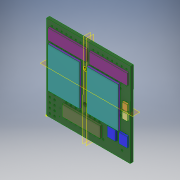
# Autodesk Inventor part: NixieModule_IN12.brd
Saved by Autodesk Inventor 2019 (Build 230136000, 136)
## iProperties
Created: 2019-08-02
Part Number: NixieModule_IN12.brd
Material: Generisch
Document SubType Name: Modeling
Designer: grubi
Density: 1 g/cm^3
Appearance: Board-Kontur
Author: grubi
Autodesk Inventor part; units mm, degrees
ref_plane "YZ Plane" through (0, 0, 0) normal (1, 0, 0) x (0, 1, 0)
ref_plane "XZ Plane" through (0, 0, 0) normal (0, 1, 0) x (-1, 0, 0)
ref_plane "XY Plane" through (0, 0, 0) normal (0, 0, 1) x (1, 0, 0)
sketch "Skizze1" plane through (0, 0, 0) normal (0, 0, 1) x (1, 0, 0)
  line L0 (0, 0) -> (44.938, 0)
  line L1 (44.938, 0) -> (45.065, 45.39)
  line L2 (45.065, 45.39) -> (0, 45.39)
  line L3 (0, 45.39) -> (0, 0)
  circle A0 centre (16.51, 7.62) radius 0.405
  circle A1 centre (21.59, 7.62) radius 0.405
  circle A2 centre (38.1, 39.37) radius 0.405
  circle A3 centre (33.02, 39.37) radius 0.405
  circle A4 centre (16.51, 39.37) radius 0.405
  circle A5 centre (11.43, 39.37) radius 0.405
  circle A6 centre (42.93, 27.56) radius 0.405
  circle A7 centre (42.93, 25.02) radius 0.405
  circle A8 centre (42.93, 19.94) radius 0.405
  circle A9 centre (42.93, 22.48) radius 0.405
  circle A10 centre (3.05, 35.43) radius 0.405
  circle A11 centre (5.59, 35.43) radius 0.405
  circle A12 centre (8.13, 35.43) radius 0.405
  circle A13 centre (10.67, 35.43) radius 0.405
  circle A14 centre (13.21, 35.43) radius 0.405
  circle A15 centre (15.75, 35.43) radius 0.405
  circle A16 centre (18.29, 35.43) radius 0.405
  circle A17 centre (20.83, 35.43) radius 0.405
  circle A18 centre (20.83, 43.05) radius 0.405
  circle A19 centre (18.29, 43.05) radius 0.405
  circle A20 centre (15.75, 43.05) radius 0.405
  circle A21 centre (13.21, 43.05) radius 0.405
  circle A22 centre (10.67, 43.05) radius 0.405
  circle A23 centre (8.13, 43.05) radius 0.405
  circle A24 centre (5.59, 43.05) radius 0.405
  circle A25 centre (3.05, 43.05) radius 0.405
  circle A26 centre (25.15, 35.43) radius 0.405
  circle A27 centre (27.69, 35.43) radius 0.405
  circle A28 centre (30.23, 35.43) radius 0.405
  circle A29 centre (32.77, 35.43) radius 0.405
  circle A30 centre (35.31, 35.43) radius 0.405
  circle A31 centre (37.85, 35.43) radius 0.405
  circle A32 centre (40.39, 35.43) radius 0.405
  circle A33 centre (42.93, 35.43) radius 0.405
  circle A34 centre (42.93, 43.05) radius 0.405
  circle A35 centre (40.39, 43.05) radius 0.405
  circle A36 centre (37.85, 43.05) radius 0.405
  circle A37 centre (35.31, 43.05) radius 0.405
  circle A38 centre (32.77, 43.05) radius 0.405
  circle A39 centre (30.23, 43.05) radius 0.405
  circle A40 centre (27.69, 43.05) radius 0.405
  circle A41 centre (25.15, 43.05) radius 0.405
  circle A42 centre (10.67, 3.68) radius 0.405
  circle A43 centre (13.21, 3.68) radius 0.405
  circle A44 centre (15.75, 3.68) radius 0.405
  circle A45 centre (18.29, 3.68) radius 0.405
  circle A46 centre (20.83, 3.68) radius 0.405
  circle A47 centre (23.37, 3.68) radius 0.405
  circle A48 centre (25.91, 3.68) radius 0.405
  circle A49 centre (28.45, 3.68) radius 0.405
  circle A50 centre (28.45, 11.3) radius 0.405
  circle A51 centre (25.91, 11.3) radius 0.405
  circle A52 centre (23.37, 11.3) radius 0.405
  circle A53 centre (20.83, 11.3) radius 0.405
  circle A54 centre (18.29, 11.3) radius 0.405
  circle A55 centre (15.75, 11.3) radius 0.405
  circle A56 centre (13.21, 11.3) radius 0.405
  circle A57 centre (10.67, 11.3) radius 0.405
  circle A58 centre (1.78, 1.78) radius 0.51
  circle A59 centre (4.32, 1.78) radius 0.51
  circle A60 centre (1.78, 4.32) radius 0.51
  circle A61 centre (4.32, 4.32) radius 0.51
  circle A62 centre (1.78, 6.86) radius 0.51
  circle A63 centre (4.32, 6.86) radius 0.51
  circle A64 centre (1.78, 9.4) radius 0.51
  circle A65 centre (4.32, 9.4) radius 0.51
  circle A66 centre (1.78, 11.94) radius 0.51
  circle A67 centre (4.32, 11.94) radius 0.51
  circle A68 centre (1.78, 14.48) radius 0.51
  circle A69 centre (4.32, 14.48) radius 0.51
  circle A70 centre (33.02, 17.78) radius 0.45
  circle A71 centre (33.02, 27.94) radius 0.45
  circle A72 centre (12.32, 18.16) radius 0.45
  circle A73 centre (12.32, 28.32) radius 0.45
  circle A74 centre (39.75, 9.78) radius 0.45
  circle A75 centre (39.75, 19.94) radius 0.45
  circle A76 centre (39.75, 32.51) radius 0.45
  circle A77 centre (39.75, 22.35) radius 0.45
  circle A78 centre (30.48, 4.06) radius 0.45
  circle A79 centre (40.64, 4.06) radius 0.45
  circle A80 centre (36.32, 10.03) radius 0.405
  circle A81 centre (36.32, 12.57) radius 0.405
  circle A82 centre (36.32, 7.49) radius 0.405
  circle A83 centre (42.55, 10.03) radius 0.405
  circle A84 centre (42.55, 12.57) radius 0.405
  circle A85 centre (42.55, 7.49) radius 0.405
  circle A86 centre (15.72, 19.25) radius 0.55
  circle A87 centre (6.35, 15.93) radius 0.55
  circle A88 centre (4.67, 19.25) radius 0.55
  circle A89 centre (4.54, 23.75) radius 0.55
  circle A90 centre (4.67, 28.25) radius 0.55
  circle A91 centre (6.35, 31.57) radius 0.55
  circle A92 centre (10.35, 32.57) radius 0.55
  circle A93 centre (14.35, 31.57) radius 0.55
  circle A94 centre (15.72, 28.25) radius 0.55
  circle A95 centre (15.84, 23.75) radius 0.55
  circle A96 centre (14.35, 15.93) radius 0.55
  circle A97 centre (10.35, 14.93) radius 0.55
  circle A98 centre (36.54, 19.25) radius 0.55
  circle A99 centre (27.18, 15.93) radius 0.55
  circle A100 centre (25.5, 19.25) radius 0.55
  circle A101 centre (25.37, 23.75) radius 0.55
  circle A102 centre (25.5, 28.25) radius 0.55
  circle A103 centre (27.18, 31.57) radius 0.55
  circle A104 centre (31.18, 32.57) radius 0.55
  circle A105 centre (35.18, 31.57) radius 0.55
  circle A106 centre (36.54, 28.25) radius 0.55
  circle A107 centre (36.67, 23.75) radius 0.55
  circle A108 centre (35.18, 15.93) radius 0.55
  circle A109 centre (31.18, 14.93) radius 0.55
  circle A110 centre (20.7645, 32.049) radius 1
  circle A111 centre (20.7645, 15.449) radius 1
  circle A112 centre (18.2372, 20.1168) radius 0.175
  circle A113 centre (32.9946, 21.0566) radius 0.175
  circle A114 centre (7.0024, 2.9384) radius 0.175
  circle A115 centre (29.3116, 6.6548) radius 0.175
  circle A116 centre (22.2504, 26.4668) radius 0.175
  circle A117 centre (27.0256, 7.5692) radius 0.175
  circle A118 centre (18.034, 40.64) radius 0.175
  circle A119 centre (23.0378, 36.9824) radius 0.175
  circle A120 centre (7.2644, 7.0104) radius 0.175
  circle A121 centre (18.3642, 28.3464) radius 0.175
  circle A122 centre (7.366, 23.2664) radius 0.175
  circle A123 centre (12.8524, 38.2016) radius 0.175
  circle A124 centre (9.1948, 38.6588) radius 0.175
  circle A125 centre (6.604, 37.4396) radius 0.175
  circle A126 centre (34.9504, 38.9636) radius 0.175
  circle A127 centre (34.9504, 37.4396) radius 0.175
  circle A128 centre (29.6164, 28.2956) radius 0.175
  circle A129 centre (29.1592, 40.6908) radius 0.175
  circle A130 centre (37.2364, 37.2872) radius 0.175
  circle A131 centre (32.512, 37.4396) radius 0.175
  circle A132 centre (31.5976, 24.1808) radius 0.175
  circle A133 centre (17.5768, 27.6352) radius 0.175
  circle A134 centre (17.4229, 14.653) radius 0.175
  circle A135 centre (33.4264, 11.9888) radius 0.175
  circle A136 centre (27.0256, 8.636) radius 0.175
  circle A137 centre (24.8158, 15.875) radius 0.175
  circle A138 centre (25.019, 31.369) radius 0.175
  circle A139 centre (20.8534, 22.0472) radius 0.175
  circle A140 centre (41.1988, 27.3812) radius 0.175
  circle A141 centre (34.3408, 14.1224) radius 0.175
  circle A142 centre (30.8356, 17.9324) radius 0.175
  circle A143 centre (38.7604, 25.2476) radius 0.175
  circle A144 centre (2.3368, 20.3708) radius 0.175
  circle A145 centre (2.3368, 24.1808) radius 0.175
  circle A146 centre (7.8232, 27.8384) radius 0.175
  circle A147 centre (28.8036, 20.9804) radius 0.175
  circle A148 centre (16.9672, 25.2476) radius 0.175
  constraints: 149 centre point, 8 end point
extrude "NixieModule_IN12.brd_Kontur" add sketch "Skizze1" along normal blind 1.6
sketch "C050-024X044, C050-024X044_1" plane through (0, 0, 0) normal (0, 0, 1) x (1, 0, 0)
  line L0 (16.51, 6.477) -> (21.59, 6.477)
  line L1 (21.59, 6.477) -> (21.59, 8.763)
  line L2 (21.59, 8.763) -> (16.51, 8.763)
  line L3 (16.51, 8.763) -> (16.51, 6.477)
  constraints: 8 end point
extrude "C100_2" add sketch "C050-024X044, C050-024X044_1" against normal blind 1
sketch "C050-024X044, C050-024X044_3" plane through (0, 0, 0) normal (0, 0, 1) x (1, 0, 0)
  line L0 (38.1, 40.513) -> (33.02, 40.513)
  line L1 (33.02, 40.513) -> (33.02, 38.227)
  line L2 (33.02, 38.227) -> (38.1, 38.227)
  line L3 (38.1, 38.227) -> (38.1, 40.513)
  constraints: 8 end point
extrude "C101_4" add sketch "C050-024X044, C050-024X044_3" against normal blind 1
sketch "C050-024X044, C050-024X044_5" plane through (0, 0, 0) normal (0, 0, 1) x (1, 0, 0)
  line L0 (16.51, 40.513) -> (11.43, 40.513)
  line L1 (11.43, 40.513) -> (11.43, 38.227)
  line L2 (11.43, 38.227) -> (16.51, 38.227)
  line L3 (16.51, 38.227) -> (16.51, 40.513)
  constraints: 8 end point
extrude "C102_6" add sketch "C050-024X044, C050-024X044_5" against normal blind 1
sketch "WS2812B, SK6812_7" plane through (0, 0, 1.6) normal (0, 0, 1) x (1, 0, 0)
  line L0 (7.2898, 26.8097) -> (12.914, 26.8097)
  line L1 (12.914, 26.8097) -> (12.914, 21.1328)
  line L2 (12.914, 21.1328) -> (7.2898, 21.1328)
  line L3 (7.2898, 21.1328) -> (7.2898, 26.8097)
  constraints: 8 end point
extrude "D1_8" add sketch "WS2812B, SK6812_7" along normal blind 1
sketch "WS2812B, SK6812_9" plane through (0, 0, 1.6) normal (0, 0, 1) x (1, 0, 0)
  line L0 (28.1178, 26.8097) -> (33.742, 26.8097)
  line L1 (33.742, 26.8097) -> (33.742, 21.1328)
  line L2 (33.742, 21.1328) -> (28.1178, 21.1328)
  line L3 (28.1178, 21.1328) -> (28.1178, 26.8097)
  constraints: 8 end point
extrude "D2_10" add sketch "WS2812B, SK6812_9" along normal blind 1
sketch "LED_LD260, GLOW1_LED_LD260_11" plane through (0, 0, 1.6) normal (0, 0, 1) x (1, 0, 0)
  line L0 (44.2722, 27.6352) -> (44.2722, 24.257)
  line L1 (44.2722, 24.257) -> (41.5798, 24.257)
  line L2 (41.5798, 24.257) -> (41.5798, 27.6352)
  line L3 (41.5798, 27.6352) -> (44.2722, 27.6352)
  constraints: 8 end point
extrude "GLOW1_12" add sketch "LED_LD260, GLOW1_LED_LD260_11" along normal blind 1
sketch "LED_LD260, GLOW2_LED_LD260_13" plane through (0, 0, 1.6) normal (0, 0, 1) x (1, 0, 0)
  line L0 (41.5798, 19.8628) -> (41.5798, 23.241)
  line L1 (41.5798, 23.241) -> (44.2722, 23.241)
  line L2 (44.2722, 23.241) -> (44.2722, 19.8628)
  line L3 (44.2722, 19.8628) -> (41.5798, 19.8628)
  constraints: 8 end point
extrude "GLOW2_14" add sketch "LED_LD260, GLOW2_LED_LD260_13" along normal blind 1
sketch "DIL16, IC_74141-DIP-16_15" plane through (0, 0, 1.6) normal (0, 0, 1) x (1, 0, 0)
  line L0 (1.7018, 42.2402) -> (22.1742, 42.2402)
  line L1 (22.1742, 42.2402) -> (22.1742, 36.322)
  line L2 (22.1742, 36.322) -> (1.7018, 36.322)
  line L3 (1.7018, 36.322) -> (1.7018, 42.2402)
  constraints: 8 end point
extrude "IC1_16" add sketch "DIL16, IC_74141-DIP-16_15" along normal blind 1
sketch "DIL16, IC_74141-DIP-16_17" plane through (0, 0, 1.6) normal (0, 0, 1) x (1, 0, 0)
  line L0 (23.7998, 42.2402) -> (44.2722, 42.2402)
  line L1 (44.2722, 42.2402) -> (44.2722, 36.322)
  line L2 (44.2722, 36.322) -> (23.7998, 36.322)
  line L3 (23.7998, 36.322) -> (23.7998, 42.2402)
  constraints: 8 end point
extrude "IC2_18" add sketch "DIL16, IC_74141-DIP-16_17" along normal blind 1
sketch "DIL16, 74LS595N_19" plane through (0, 0, 1.6) normal (0, 0, 1) x (1, 0, 0)
  line L0 (9.3218, 10.4902) -> (29.7942, 10.4902)
  line L1 (29.7942, 10.4902) -> (29.7942, 4.572)
  line L2 (29.7942, 4.572) -> (9.3218, 4.572)
  line L3 (9.3218, 4.572) -> (9.3218, 10.4902)
  constraints: 8 end point
extrude "IC3_20" add sketch "DIL16, 74LS595N_19" along normal blind 1
sketch "MA06-2, MA06-2_21" plane through (0, 0, 0) normal (0, 0, 1) x (1, 0, 0)
  line L0 (5.6642, 0.508) -> (5.6642, 15.748)
  line L1 (5.6642, 15.748) -> (0.508, 15.748)
  line L2 (0.508, 15.748) -> (0.508, 0.508)
  line L3 (0.508, 0.508) -> (5.6642, 0.508)
  constraints: 8 end point
extrude "NIXIE_22" add sketch "MA06-2, MA06-2_21" against normal blind 1
sketch "AXIAL-0_4, R_AN100_AXIAL-0_4_23" plane through (0, 0, 0) normal (0, 0, 1) x (1, 0, 0)
  line L0 (34.3216, 19.6084) -> (34.3216, 26.01)
  line L1 (34.3216, 26.01) -> (31.7184, 26.01)
  line L2 (31.7184, 26.01) -> (31.7184, 19.6084)
  line L3 (31.7184, 19.6084) -> (34.3216, 19.6084)
  constraints: 8 end point
extrude "R_AN100_24" add sketch "AXIAL-0_4, R_AN100_AXIAL-0_4_23" against normal blind 1
sketch "AXIAL-0_4, R_AN101_AXIAL-0_4_25" plane through (0, 0, 0) normal (0, 0, 1) x (1, 0, 0)
  line L0 (13.6206, 19.9894) -> (13.6206, 26.391)
  line L1 (13.6206, 26.391) -> (11.0174, 26.391)
  line L2 (11.0174, 26.391) -> (11.0174, 19.9894)
  line L3 (11.0174, 19.9894) -> (13.6206, 19.9894)
  constraints: 8 end point
extrude "R_AN101_26" add sketch "AXIAL-0_4, R_AN101_AXIAL-0_4_25" against normal blind 1
sketch "AXIAL-0_4, R_AN_COL100_AXIAL-0_4_27" plane through (0, 0, 0) normal (0, 0, 1) x (1, 0, 0)
  line L0 (41.0526, 11.6074) -> (41.0526, 18.009)
  line L1 (41.0526, 18.009) -> (38.4494, 18.009)
  line L2 (38.4494, 18.009) -> (38.4494, 11.6074)
  line L3 (38.4494, 11.6074) -> (41.0526, 11.6074)
  constraints: 8 end point
extrude "R_AN_COL100_28" add sketch "AXIAL-0_4, R_AN_COL100_AXIAL-0_4_27" against normal blind 1
sketch "AXIAL-0_4, R_AN_COL101_AXIAL-0_4_29" plane through (0, 0, 0) normal (0, 0, 1) x (1, 0, 0)
  line L0 (38.4494, 30.6836) -> (38.4494, 24.282)
  line L1 (38.4494, 24.282) -> (41.0526, 24.282)
  line L2 (41.0526, 24.282) -> (41.0526, 30.6836)
  line L3 (41.0526, 30.6836) -> (38.4494, 30.6836)
  constraints: 8 end point
extrude "R_AN_COL101_30" add sketch "AXIAL-0_4, R_AN_COL101_AXIAL-0_4_29" against normal blind 1
sketch "AXIAL-0_4, R_BASE_AXIAL-0_4_31" plane through (0, 0, 0) normal (0, 0, 1) x (1, 0, 0)
  line L0 (32.3084, 2.7624) -> (38.71, 2.7624)
  line L1 (38.71, 2.7624) -> (38.71, 5.3656)
  line L2 (38.71, 5.3656) -> (32.3084, 5.3656)
  line L3 (32.3084, 5.3656) -> (32.3084, 2.7624)
  constraints: 8 end point
extrude "R_BASE_32" add sketch "AXIAL-0_4, R_BASE_AXIAL-0_4_31" against normal blind 1
sketch "TO92-EBC, TO92-EBC_33" plane through (0, 0, 1.6) normal (0, 0, 1) x (1, 0, 0)
  line L0 (33.5915, 7.3025) -> (33.5915, 12.7)
  line L1 (33.5915, 12.7) -> (38.0365, 12.7)
  line L2 (38.0365, 12.7) -> (38.0365, 7.3025)
  line L3 (38.0365, 7.3025) -> (33.5915, 7.3025)
  constraints: 8 end point
extrude "T1_34" add sketch "TO92-EBC, TO92-EBC_33" along normal blind 1
sketch "TO92-EBC, TO92-EBC_35" plane through (0, 0, 1.6) normal (0, 0, 1) x (1, 0, 0)
  line L0 (39.8145, 7.3025) -> (39.8145, 12.7)
  line L1 (39.8145, 12.7) -> (44.2595, 12.7)
  line L2 (44.2595, 12.7) -> (44.2595, 7.3025)
  line L3 (44.2595, 7.3025) -> (39.8145, 7.3025)
  constraints: 8 end point
extrude "T2_36" add sketch "TO92-EBC, TO92-EBC_35" along normal blind 1
sketch "IN-12, IN-12A_37" plane through (0, 0, 1.6) normal (0, 0, 1) x (1, 0, 0)
  line L0 (1.7145, 34.6653) -> (18.669, 34.6653)
  line L1 (18.669, 34.6653) -> (18.669, 12.8504)
  line L2 (18.669, 12.8504) -> (1.7145, 12.8504)
  line L3 (1.7145, 12.8504) -> (1.7145, 34.6653)
  constraints: 8 end point
extrude "TUBE-1_38" add sketch "IN-12, IN-12A_37" along normal blind 1
sketch "IN-12, IN-12A_39" plane through (0, 0, 1.6) normal (0, 0, 1) x (1, 0, 0)
  line L0 (22.5425, 34.6653) -> (39.497, 34.6653)
  line L1 (39.497, 34.6653) -> (39.497, 12.8504)
  line L2 (39.497, 12.8504) -> (22.5425, 12.8504)
  line L3 (22.5425, 12.8504) -> (22.5425, 34.6653)
  constraints: 8 end point
extrude "TUBE-2_40" add sketch "IN-12, IN-12A_39" along normal blind 1
ref_plane "Arbeitsebene1" through (0, -16060.912, 1.6) normal (1, -0.0014, 0) x (0, 0, 1)
sketch "Skizze22" plane through (0, 0, 1.6) normal (0, 0, 1) x (1, 0, 0)
  circle A0 centre (20.7645, 32.049) radius 1 projected
  point P0 (0, 0)
ref_plane "Arbeitsebene2" through (20.7645, 32.049, 1.6) normal (1, -0.0014, 0) x (0, 0, 1)
sketch "Skizze25" plane through (0, 0, 0) normal (0, 0, -1) x (-1, 0, 0)
  circle A0 centre (-25.37, 23.75) radius 0.55 projected
  point P0 (0, 0)
ref_plane "Arbeitsebene4" through (25.37, 23.75, 0) normal (0, 1, 0) x (1, 0, 0)
